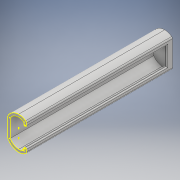
# Autodesk Inventor part: obudowa
Saved by Autodesk Inventor 2017 (Build 210142000, 142)
## iProperties
Created: 2019-10-26
Part Number: obudowa
Material: Ogólny
Document SubType Name: Modeling
Designer: patry
Density: 1 g/cm^3
Appearance: Domyślna
Author: patry
Autodesk Inventor part; units mm, degrees
ref_plane "YZ Plane" through (0, 0, 0) normal (1, 0, 0) x (0, 1, 0)
ref_plane "XZ Plane" through (0, 0, 0) normal (0, 1, 0) x (-1, 0, 0)
ref_plane "XY Plane" through (0, 0, 0) normal (0, 0, 1) x (1, 0, 0)
sketch "Szkic1" plane through (0, 0, 0) normal (0, 1, 0) x (-1, 0, 0)
  spline S0 degree 3 poles (4.29, 24.6442) (4.4521, 24.6442) (4.6114, 24.6406) (4.7677, 24.6336) (4.8034, 24.632) (4.8389, 24.6302) (4.8743, 24.6283) (4.9939, 24.6216) (5.1117, 24.613) (5.2279, 24.6025) (5.2909, 24.5968) (5.3533, 24.5906) (5.4152, 24.5838) (5.5016, 24.5743) (5.5869, 24.5637) (5.6714, 24.5521) (5.7603, 24.5399) (5.8483, 24.5266) (5.9352, 24.5122) (5.9902, 24.503) (6.0448, 24.4934) (6.099, 24.4834) (6.213, 24.4624) (6.3254, 24.4394) (6.4363, 24.4145) (6.4615, 24.4088) (6.4866, 24.4031) (6.5116, 24.3972) (6.6467, 24.3657) (6.7795, 24.3313) (6.9102, 24.2942) (7.0408, 24.2571) (7.1693, 24.2173) (7.2957, 24.1748) (7.3261, 24.1646) (7.3564, 24.1542) (7.3866, 24.1437) (7.4819, 24.1104) (7.576, 24.0756) (7.6691, 24.0393) (7.7261, 24.0171) (7.7827, 23.9943) (7.8389, 23.9709) (7.9035, 23.944) (7.9676, 23.9164) (8.0312, 23.888) (8.1143, 23.8509) (8.1964, 23.8125) (8.2778, 23.7729) (8.313, 23.7557) (8.348, 23.7383) (8.3829, 23.7207) (8.4915, 23.6658) (8.5987, 23.6086) (8.7045, 23.5489) (8.7113, 23.5451) (8.7181, 23.5412) (8.7249, 23.5374) (8.8374, 23.4736) (8.9484, 23.407) (9.058, 23.3376) (9.0788, 23.3245) (9.0995, 23.3112) (9.1202, 23.2979) (9.2086, 23.2408) (9.2961, 23.1819) (9.3827, 23.121) (9.4307, 23.0873) (9.4784, 23.0531) (9.5258, 23.0182) (9.5842, 22.9753) (9.6421, 22.9315) (9.6997, 22.8868) (9.7745, 22.8287) (9.8486, 22.7691) (9.9222, 22.7079) (9.9514, 22.6836) (9.9805, 22.659) (10.0095, 22.6342) (10.1116, 22.5468) (10.2126, 22.4562) (10.3125, 22.3621) (10.4124, 22.2681) (10.5112, 22.1706) (10.609, 22.0695) (10.6346, 22.043) (10.6601, 22.0163) (10.6855, 21.9894) (10.7573, 21.9132) (10.8286, 21.8351) (10.8993, 21.7548) (10.9505, 21.6966) (11.0014, 21.6374) (11.052, 21.577) (11.0961, 21.5244) (11.1399, 21.4708) (11.1836, 21.4164) (11.2594, 21.3219) (11.3345, 21.2247) (11.409, 21.1244) (11.4266, 21.1006) (11.4443, 21.0767) (11.4619, 21.0525) (11.5537, 20.9267) (11.6444, 20.7964) (11.7342, 20.661) (11.7412, 20.6503) (11.7483, 20.6396) (11.7554, 20.6289) (11.8379, 20.5035) (11.9195, 20.3738) (12, 20.2398) knots 0 0 0 0 0.045455 0.045455 0.045455 0.05583 0.05583 0.05583 0.090909 0.090909 0.090909 0.109901 0.109901 0.109901 0.136364 0.136364 0.136364 0.164215 0.164215 0.164215 0.181818 0.181818 0.181818 0.218856 0.218856 0.218856 0.227273 0.227273 0.227273 0.272727 0.272727 0.272727 0.318182 0.318182 0.318182 0.329116 0.329116 0.329116 0.363636 0.363636 0.363636 0.384782 0.384782 0.384782 0.409091 0.409091 0.409091 0.440823 0.440823 0.440823 0.454545 0.454545 0.454545 0.497251 0.497251 0.497251 0.5 0.5 0.5 0.545455 0.545455 0.545455 0.554072 0.554072 0.554072 0.590909 0.590909 0.590909 0.611291 0.611291 0.611291 0.636364 0.636364 0.636364 0.668896 0.668896 0.668896 0.681818 0.681818 0.681818 0.727273 0.727273 0.727273 0.772727 0.772727 0.772727 0.784612 0.784612 0.784612 0.818182 0.818182 0.818182 0.842477 0.842477 0.842477 0.863636 0.863636 0.863636 0.900365 0.900365 0.900365 0.909091 0.909091 0.909091 0.954545 0.954545 0.954545 0.958127 0.958127 0.958127 1 1 1 1
  spline S1 degree 3 poles (0, 23.3634) (0.0313, 23.3834) (0.0629, 23.4032) (0.0948, 23.4229) (0.1661, 23.4669) (0.2387, 23.51) (0.3127, 23.5522) (0.3366, 23.5659) (0.3606, 23.5794) (0.3848, 23.5929) (0.4689, 23.6397) (0.5548, 23.6854) (0.6428, 23.7301) (0.6619, 23.7398) (0.6811, 23.7494) (0.7004, 23.759) (0.7955, 23.8063) (0.893, 23.8524) (0.9925, 23.8971) (1.0001, 23.9005) (1.0078, 23.9039) (1.0155, 23.9073) (1.1133, 23.9508) (1.213, 23.9929) (1.3144, 24.0334) (1.3295, 24.0394) (1.3447, 24.0454) (1.3599, 24.0514) (1.4359, 24.0812) (1.5128, 24.1101) (1.5905, 24.138) (1.6407, 24.156) (1.6913, 24.1737) (1.7423, 24.1909) (1.7757, 24.2022) (1.8093, 24.2133) (1.843, 24.2243) (1.9195, 24.2491) (1.9968, 24.2731) (2.0748, 24.2961) (2.096, 24.3023) (2.1174, 24.3085) (2.1387, 24.3146) (2.1887, 24.3289) (2.2389, 24.3428) (2.2893, 24.3563) (2.3554, 24.374) (2.4218, 24.391) (2.4885, 24.4072) (2.5077, 24.4119) (2.527, 24.4165) (2.5463, 24.4211) (2.5883, 24.431) (2.6305, 24.4407) (2.6727, 24.45) (2.7293, 24.4625) (2.786, 24.4745) (2.8426, 24.4858) (2.8813, 24.4936) (2.9201, 24.5011) (2.9588, 24.5084) (2.9723, 24.5109) (2.9859, 24.5134) (2.9995, 24.5159) (3.0482, 24.5248) (3.0967, 24.5332) (3.1446, 24.5411) (3.1899, 24.5486) (3.2347, 24.5556) (3.2786, 24.5621) (3.3055, 24.5661) (3.332, 24.57) (3.3581, 24.5736) (3.373, 24.5757) (3.3878, 24.5777) (3.4024, 24.5797) (3.4415, 24.5849) (3.4798, 24.5898) (3.5172, 24.5942) (3.5534, 24.5986) (3.5889, 24.6026) (3.6237, 24.6062) (3.6534, 24.6094) (3.6826, 24.6123) (3.7112, 24.615) (3.7155, 24.6154) (3.7198, 24.6158) (3.724, 24.6162) (3.7577, 24.6193) (3.7907, 24.6221) (3.823, 24.6246) (3.8575, 24.6273) (3.8912, 24.6297) (3.9242, 24.6318) (3.9568, 24.6339) (3.9888, 24.6357) (4.0201, 24.6372) (4.0561, 24.639) (4.0912, 24.6404) (4.1254, 24.6415) (4.1561, 24.6425) (4.186, 24.6432) (4.2153, 24.6436) (4.2407, 24.644) (4.2656, 24.6442) (4.29, 24.6442) knots 0 0 0 0 0.025747 0.025747 0.025747 0.083333 0.083333 0.083333 0.101932 0.101932 0.101932 0.166667 0.166667 0.166667 0.180728 0.180728 0.180728 0.25 0.25 0.25 0.255325 0.255325 0.255325 0.323187 0.323187 0.323187 0.333333 0.333333 0.333333 0.383956 0.383956 0.383956 0.416667 0.416667 0.416667 0.438102 0.438102 0.438102 0.486742 0.486742 0.486742 0.5 0.5 0.5 0.531015 0.531015 0.531015 0.571623 0.571623 0.571623 0.583333 0.583333 0.583333 0.608888 0.608888 0.608888 0.643164 0.643164 0.643164 0.666667 0.666667 0.666667 0.674925 0.674925 0.674925 0.704638 0.704638 0.704638 0.732781 0.732781 0.732781 0.75 0.75 0.75 0.759817 0.759817 0.759817 0.786075 0.786075 0.786075 0.811555 0.811555 0.811555 0.833333 0.833333 0.833333 0.836565 0.836565 0.836565 0.86226 0.86226 0.86226 0.889614 0.889614 0.889614 0.916667 0.916667 0.916667 0.947785 0.947785 0.947785 0.975695 0.975695 0.975695 1 1 1 1
  line L0 (0, 23.3634) -> (0, 0)
  spline S2 degree 3 poles (4.29, -1.2808) (4.2555, -1.2808) (4.2199, -1.2804) (4.1832, -1.2796) (4.15, -1.2789) (4.1159, -1.2779) (4.081, -1.2765) (4.0607, -1.2757) (4.0401, -1.2748) (4.0192, -1.2737) (4.0064, -1.2731) (3.9935, -1.2724) (3.9804, -1.2717) (3.948, -1.2699) (3.9149, -1.2678) (3.881, -1.2655) (3.8471, -1.2631) (3.8125, -1.2604) (3.7771, -1.2574) (3.7548, -1.2555) (3.7322, -1.2535) (3.7093, -1.2513) (3.6944, -1.2499) (3.6793, -1.2485) (3.664, -1.2469) (3.6238, -1.2429) (3.5825, -1.2385) (3.5402, -1.2335) (3.496, -1.2284) (3.4506, -1.2227) (3.4039, -1.2164) (3.3878, -1.2143) (3.3716, -1.2121) (3.3552, -1.2098) (3.322, -1.2051) (3.2881, -1.2002) (3.2538, -1.1949) (3.1998, -1.1867) (3.1445, -1.1778) (3.0886, -1.1682) (3.0444, -1.1606) (2.9999, -1.1526) (2.9552, -1.1443) (2.9389, -1.1412) (2.9225, -1.1381) (2.9062, -1.1349) (2.8392, -1.122) (2.7721, -1.1082) (2.7051, -1.0937) (2.6511, -1.0819) (2.5971, -1.0696) (2.5432, -1.0569) (2.5237, -1.0523) (2.5042, -1.0476) (2.4847, -1.0428) (2.4029, -1.0229) (2.3215, -1.0019) (2.2408, -0.9798) (2.2058, -0.9702) (2.1709, -0.9604) (2.1362, -0.9505) (2.0792, -0.9341) (2.0226, -0.9173) (1.9664, -0.8999) (1.8903, -0.8764) (1.8149, -0.8521) (1.7404, -0.8268) (1.7134, -0.8177) (1.6866, -0.8084) (1.6598, -0.7991) (1.5579, -0.7635) (1.4574, -0.7262) (1.3585, -0.6874) (1.3491, -0.6837) (1.3397, -0.68) (1.3303, -0.6762) (1.2151, -0.6306) (1.102, -0.5828) (0.9914, -0.5331) (0.8892, -0.4873) (0.7891, -0.4398) (0.6916, -0.3912) (0.675, -0.3829) (0.6585, -0.3746) (0.642, -0.3662) (0.5634, -0.3263) (0.4865, -0.2856) (0.4111, -0.244) (0.3779, -0.2257) (0.3451, -0.2073) (0.3125, -0.1887) (0.2537, -0.1551) (0.1957, -0.1209) (0.1385, -0.0862) (0.0918, -0.0578) (0.0456, -0.0291) (0, 0) knots 0 0 0 0 0.034308 0.034308 0.034308 0.065329 0.065329 0.065329 0.083333 0.083333 0.083333 0.094376 0.094376 0.094376 0.121838 0.121838 0.121838 0.149346 0.149346 0.149346 0.166667 0.166667 0.166667 0.177988 0.177988 0.177988 0.207919 0.207919 0.207919 0.239209 0.239209 0.239209 0.25 0.25 0.25 0.271822 0.271822 0.271822 0.306177 0.306177 0.306177 0.333333 0.333333 0.333333 0.343269 0.343269 0.343269 0.383905 0.383905 0.383905 0.416667 0.416667 0.416667 0.428546 0.428546 0.428546 0.478409 0.478409 0.478409 0.5 0.5 0.5 0.535413 0.535413 0.535413 0.583333 0.583333 0.583333 0.60065 0.60065 0.60065 0.666667 0.666667 0.666667 0.672941 0.672941 0.672941 0.75 0.75 0.75 0.821219 0.821219 0.821219 0.833333 0.833333 0.833333 0.891251 0.891251 0.891251 0.916667 0.916667 0.916667 0.962519 0.962519 0.962519 1 1 1 1
  spline S3 degree 3 poles (12, 3.1236) (11.9126, 2.9781) (11.7351, 2.6973) (11.4629, 2.3063) (11.1845, 1.9427) (10.9003, 1.6047) (10.61, 1.2902) (10.3135, 0.9978) (10.0106, 0.726) (9.7008, 0.4735) (9.3839, 0.2395) (9.0593, 0.0229) (8.7263, -0.1767) (8.3844, -0.36) (8.0328, -0.5272) (7.6709, -0.6786) (7.2976, -0.814) (6.9122, -0.9335) (6.5138, -1.0366) (6.1013, -1.1229) (5.674, -1.1918) (5.2306, -1.2423) (4.7705, -1.2736) (4.4521, -1.2808) (4.29, -1.2808) knots 0 0 0 0 0.045455 0.090909 0.136364 0.181818 0.227273 0.272727 0.318182 0.363636 0.409091 0.454545 0.5 0.545455 0.590909 0.636364 0.681818 0.727273 0.772727 0.818182 0.863636 0.909091 0.954545 1 1 1 1
  line L1 (12, 3.1236) -> (12, 20.2398)
  line L2 (15.25, 21.068) -> (15.25, 2.2955)
  line L3 (-3.25, 24.9608) -> (-3.25, -1.5975)
  line L4 (12.75, 20.4434) -> (12.75, 2.92)
  line L5 (-0.75, 23.7632) -> (-0.75, -0.3998)
  arc A0 (4.29, -2.0308) -> (12.75, 2.92) centre (4.2141, 7.8027) ccw
  arc A1 (-0.75, -0.3998) -> (4.29, -2.0308) centre (4.3944, 6.8945) ccw
  line L6 (0, 0) -> (-0.4031, -0.6325) construction
  line L7 (12, 3.1236) -> (12.6428, 2.7373) construction
  arc A2 (12.75, 20.4434) -> (4.29, 25.3942) centre (4.2141, 15.5608) ccw
  arc A3 (4.29, 25.3942) -> (-0.75, 23.7632) centre (4.3942, 16.4697) ccw
  line L8 (12, 20.2398) -> (12.6428, 20.6262) construction
  line L9 (0, 23.3634) -> (-0.4031, 23.9959) construction
  arc A4 (4.29, -4.5308) -> (15.25, 2.2955) centre (4.2142, 7.8026) ccw
  arc A5 (-3.25, -1.5975) -> (4.29, -4.5308) centre (4.394, 6.8939) ccw
  arc A6 (15.25, 21.068) -> (4.29, 27.8942) centre (4.2142, 15.5608) ccw
  arc A7 (4.29, 27.8942) -> (-3.25, 24.9608) centre (4.3938, 16.4703) ccw
  line L10 (12.6428, 2.7373) -> (14.7857, 1.4495) construction
  line L11 (12.75, 20.4434) -> (14.9201, 21.6847) construction
  line L12 (-0.75, 23.7632) -> (-2.1909, 25.8062) construction
  line L13 (-0.75, -0.3998) -> (-2.1909, -2.4428) construction
  line L14 (-0.75, 2.6002) -> (-3.25, 2.6002)
  line L15 (-0.75, 20.7632) -> (-3.25, 20.7632)
  point P0 (0, 0)
  point P1 (0, 11.6817)
  dimension "d8" = 0.75
  dimension "d9" = 0.75
  dimension "d14" = 0.75
  dimension "d15" = 0.75
  dimension "d16" = 0.75
  dimension "d17" = 0.75
  dimension "d18" = 0.75
  dimension "d19" = 0.75
  dimension "d20" = 2.5
  dimension "d21" = 2.5
  dimension "d22" = 2.5
  dimension "d23" = 2.5
  dimension "d24" = 2.5
  dimension "d25" = 2.5
  dimension "d26" = 2.5
  dimension "d28" = 2.5
  dimension "d29" = 3
  dimension "d30" = 3
  constraints: 32 end point, 24 point on circle, 12 line through centre, 8 centre point, 4 point on line, 4 vertical, 4 vertical alignment, 2 parallel, 2 perpendicular, 24 other
  measures "d8" distance between parallel lines of L0 L5
  measures "d9" distance from line of L1.start L4
  measures "d14" distance of point (4.29, -1.281) A0.start
  measures "d15" distance of L0.end L6.end
  measures "d16" distance of L1.start L7.end
  measures "d17" distance of point (4.29, 24.644) A2.end
  measures "d18" distance of L1.end L8.end
  measures "d19" distance of L0.start L9.end
  measures "d20" distance between parallel lines of L2 L4
  measures "d21" distance between parallel lines of L5 L3
  measures "d22" distance of A4.start A0.start
  measures "d23" distance of A2.end A6.end
  measures "d24" distance of L7.end L10.end
  measures "d25" distance of L4.start L11.end
  measures "d26" distance of L5.start L12.end
  measures "d28" distance of L5.end L13.end
  measures "d29" distance from line of L14 L5.end
  measures "d30" distance from line of L15 L5.start
extrude "Wyciągnięcie proste2" add sketch "Szkic1" along normal blind 2.5 contours S0 L1 S3 S2 L0 S1 | L2 A4 A5 L3 L14 L5 A1 A0 L4 A2 A3 L15 A7 A6 | L15 L5 L14 L3 | L5 A3 A2 L4 A0 A1
extrude "Wyciągnięcie proste3" add sketch "Szkic1" against normal blind 3 contours L15 L5 L14 L3
extrude "Wyciągnięcie proste4" add sketch "Szkic1" against normal blind 141.5 contours L2 A4 A5 L3 L14 L5 A1 A0 L4 A2 A3 L15 A7 A6
fillet "Zaokrąglenie1" radius 1 6 edges at (3.25, -72.25, 20.7632) (3.25, -72.25, 2.6002) (0.75, -72.25, 2.6002) (0.75, -72.25, 20.7632) (0.75, -3, 11.6817) (3.25, -3, 11.6817)
fillet "Zaokrąglenie2" radius 2 4 edges at (3.25, -69.5, 24.9608) (3.25, -69.5, -1.5975) (-15.25, -69.5, 2.2955) (-15.25, -69.5, 21.068)
sketch "Szkic2" plane through (-15.25, -141.5, 20.5746) normal (-1, 0, 0) x (0, 0, 1)
  line L0 (0, 144) -> (0, 0) projected
  line L1 (-17.7857, 144) -> (0, 144) projected
  line L2 (-17.7857, 0) -> (-17.7857, 144) projected
  line L3 (0, 0) -> (-17.7857, 0) projected
  line L4 (-0.1311, 141.5) -> (-17.6546, 141.5) projected
  point P0 (-20.5746, 141.5)
  point P1 (-8.8929, 70.75)
  point P2 (-8.8929, 95.75)
  point P3 (-8.8929, 45.75)
  dimension "d39" = 70.75
  dimension "d40" = 8.8929
  dimension "d41" = 17.7857
  dimension "d42" = 25
  dimension "d43" = 50
  constraints: 2 vertical alignment
  measures "d39" distance from line of L4 point (-8.893, 70.75)
  measures "d40" distance from line of L0 point (-8.893, 70.75)
  measures "d41" distance between parallel lines of L0 L2
  measures "d42" distance of point (-8.893, 70.75) point (-8.893, 45.75)
  measures "d43" distance of point (-8.893, 45.75) point (-8.893, 95.75)
hole "Otwór1" at (-15.25, -45.75, 11.6817) at (-15.25, -95.75, 11.6817) direction (1, 0, 0) diameter 3.9 depth 8 tip angle 118 clearance for "Śruba ze łbem płaskim obrobiona" size "M3.5" standard "ANSI Profil metryczny M"
sketch "Szkic3" plane through (0, -141.5, 0) normal (0, -1, 0) x (1, 0, 0)
  arc A0 (-4.29, 25.3942) -> (-12.75, 20.4434) centre (-4.2141, 15.5608) ccw projected
  arc A1 (-4.29, 27.8942) -> (-14.9988, 21.545) centre (-4.2142, 15.5608) ccw projected
  arc A2 (-14.9988, 21.545) -> (-15.25, 20.5746) centre (-13.25, 20.5746) ccw projected
  line L0 (-15.25, 20.5746) -> (-15.25, 2.7889) projected
  arc A3 (-15.25, 2.7889) -> (-14.9988, 1.8185) centre (-13.25, 2.7889) ccw projected
  arc A4 (-14.9988, 1.8185) -> (-4.29, -4.5308) centre (-4.2142, 7.8026) ccw projected
  arc A5 (-4.29, -4.5308) -> (2.4476, -2.2563) centre (-4.394, 6.8939) ccw projected
  arc A6 (2.4476, -2.2563) -> (3.25, -0.6545) centre (1.25, -0.6545) ccw projected
  line L1 (3.25, -0.6545) -> (3.25, 1.6002) projected
  arc A7 (3.25, 1.6002) -> (2.25, 2.6002) centre (2.25, 1.6002) ccw projected
  line L2 (2.25, 2.6002) -> (1.75, 2.6002) projected
  arc A8 (1.75, 2.6002) -> (0.75, 1.6002) centre (1.75, 1.6002) ccw projected
  line L3 (0.75, 1.6002) -> (0.75, -0.3998) projected
  arc A9 (-4.29, -2.0308) -> (0.75, -0.3998) centre (-4.3944, 6.8945) ccw projected
  arc A10 (-12.75, 2.92) -> (-4.29, -2.0308) centre (-4.2141, 7.8027) ccw projected
  line L4 (-12.75, 2.92) -> (-12.75, 20.4434) projected
  arc A11 (-4.29, 25.3942) -> (-12.75, 20.4434) centre (-4.2141, 15.5608) ccw projected
  arc A12 (0.75, 23.7632) -> (-4.29, 25.3942) centre (-4.3942, 16.4697) ccw projected
  line L5 (0.75, 23.7632) -> (0.75, 21.7632) projected
  arc A13 (0.75, 21.7632) -> (1.75, 20.7632) centre (1.75, 21.7632) ccw projected
  line L6 (1.75, 20.7632) -> (2.25, 20.7632) projected
  arc A14 (2.25, 20.7632) -> (3.25, 21.7632) centre (2.25, 21.7632) ccw projected
  line L7 (3.25, 21.7632) -> (3.25, 24.0179) projected
  arc A15 (3.25, 24.0179) -> (2.4477, 25.6197) centre (1.25, 24.0179) ccw projected
  arc A16 (2.4477, 25.6197) -> (-4.29, 27.8942) centre (-4.3938, 16.4703) ccw projected
  arc A17 (-4.29, 27.8942) -> (-14.9988, 21.545) centre (-4.2142, 15.5608) ccw projected
  point P0 (0, 0)
equation "\"d8\" = blad_kurczenia"
equation "\"d9\" = d8"
equation "\"d14\" = d9"
equation "\"d15\" = d8"
equation "\"d16\" = d9"
equation "\"d17\" = d14"
equation "\"d18\" = d17"
equation "\"d19\" = d17"
equation "\"d20\" = gr_scianki"
equation "\"d21\" = d20"
equation "\"d22\" = d20"
equation "\"d23\" = d21"
equation "\"d24\" = d20"
equation "\"d25\" = d21"
equation "\"d26\" = d23"
equation "\"d28\" = d22"
equation "\"d29\" = dlg_ogranicznikowi"
equation "\"d30\" = d29"
equation "\"d31\" = gr_scianki"
equation "\"d33\" = dlg_ogranicznikowi"
equation "\"d35\" = dlg_kamery + 2 * blad_kurczenia"
equation "\"d39\" = 0.5 * dlg_kamery + blad_kurczenia"
equation "\"d40\" = 0.5 * d41"
equation "\"d42\" = 0.5 * d43"
equation "\"d43\" = rozstaw_otw"
equation "\"gr_scianki\" = 2.5"
equation "\"blad_kurczenia\" = 0.75"
equation "\"dlg_ogranicznikowi\" = 3"
equation "\"rozstaw_otw\" = 50"
equation "\"dlg_kamery\" = 140"
